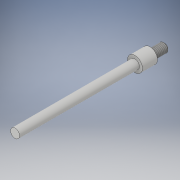
# Autodesk Inventor part: piston_axe
Saved by Autodesk Inventor 2019 (Build 230136000, 136)
## iProperties
Created: 2019-03-19
Part Number: piston_axe
Material: Générique
Document SubType Name: Modeling
Designer: theor
Density: 1 g/cm^3
Appearance: Par défaut
Author: theor
Autodesk Inventor part; units mm, degrees
ref_plane "YZ Plane" through (0, 0, 0) normal (1, 0, 0) x (0, 1, 0)
ref_plane "XZ Plane" through (0, 0, 0) normal (0, 1, 0) x (-1, 0, 0)
ref_plane "XY Plane" through (0, 0, 0) normal (0, 0, 1) x (1, 0, 0)
sketch "Esquisse2" plane through (0, 0, 0) normal (1, 0, 0) x (0, 1, 0)
  line L0 (0, 0) -> (0, -2.1683)
  line L1 (0, 0) -> (0, 50)
  line L2 (0, 0) -> (1.5, 0)
  line L3 (1.5, 0) -> (1.5, 5)
  line L4 (1.5, 5) -> (2.5, 5)
  line L5 (2.5, 5) -> (2.5, 10)
  line L6 (2.5, 10) -> (1.5, 10)
  line L7 (1.5, 10) -> (1.5, 50)
  line L8 (0, 50) -> (1.5, 50)
  dimension "d0" = 3
  dimension "d1" = 1
  dimension "d2" = 5
  dimension "d3" = 5
  dimension "d4" = 40
  constraints: 18 end point, 5 vertical, 4 horizontal, 1 collinear
  measures "d0" diameter of L3 L0
  measures "d1" distance between parallel lines of L5 L7
  measures "d2" distance between parallel lines of L2 L4
  measures "d3" distance between parallel lines of L4 L6
  measures "d4" distance between parallel lines of L8 L6
revolve "Révolution1" add sketch "Esquisse2" angle 360 about axis through (0, 0, 0) along (0, 0, -1)
thread "Filetage1" size "M3x0.5" class "6g" standard "ISO Metric profile" full length
chamfer "Chanfrein1" distance 0.5 angle 45 1 edges at (0, -1.5, 0)
